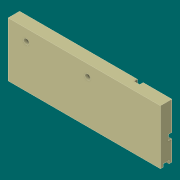
# Autodesk Inventor part: sensorHolder
Saved by Autodesk Inventor 2016 (Build 200138000, 138)
## iProperties
Created: 2015-10-19
Part Number: sensorHolder
Material: ABS Plastic
Document SubType Name: Modeling
Designer: Sawaiz
Density: 1.06 g/cm^3
Appearance: Smooth - Ash
Author: Sawaiz
Autodesk Inventor part; units mm, degrees
ref_plane "YZ Plane" through (0, 0, 0) normal (1, 0, 0) x (0, 1, 0)
ref_plane "XZ Plane" through (0, 0, 0) normal (0, 1, 0) x (-1, 0, 0)
ref_plane "XY Plane" through (0, 0, 0) normal (0, 0, 1) x (1, 0, 0)
sketch "Sketch1" plane through (0, 0, 0) normal (1, 0, 0) x (0, 1, 0)
  line L0 (-57.15, 57.15) -> (57.15, 57.15)
  line L1 (57.15, 57.15) -> (57.15, 0)
  line L2 (57.15, 0) -> (-57.15, 0)
  line L3 (-57.15, 0) -> (-57.15, 57.15)
  line L4 (-57.15, 57.15) -> (57.15, 0) construction
  line L5 (57.15, 57.15) -> (-57.15, 0) construction
  line L6 (-26.9875, 0) -> (26.9875, 0)
  line L7 (26.9875, 0) -> (26.9875, 26.9875)
  line L8 (26.9875, 26.9875) -> (-26.9875, 26.9875)
  line L9 (-26.9875, 26.9875) -> (-26.9875, 0)
  line L10 (-26.9875, 26.9875) -> (-26.9875, 57.15)
  line L11 (26.9875, 26.9875) -> (57.15, 26.9875)
  point P0 (0, 0)
  point P1 (0, 28.575)
  point P2 (0, 0)
  dimension "d5" = 114.3
  dimension "d6" = 57.15
  dimension "d7" = 53.975
  dimension "d8" = 26.9875
  constraints: 24 end point, 4 midpoint, 4 parallel, 3 horizontal, 3 point on line, 2 perpendicular, 1 coincident, 1 vertical
  measures "d5" distance between parallel lines of L3 L1
  measures "d6" distance of L0.end L1.end
  measures "d7" distance of L7.end L8.end
  measures "d8" distance of L6.end L7.end
extrude "Extrusion1" add sketch "Sketch1" along normal blind 6.35 contours L0 L1 L11 L8 L10
sketch "Sketch2" plane through (0, -26.9875, 26.9875) normal (0, 0, -1) x (-1, 0, 0)
  line L0 (0, 0) -> (0, 84.1375) projected
  line L1 (0, 84.1375) -> (-6.35, 84.1375) projected
  line L2 (-6.35, 0) -> (-6.35, 84.1375) projected
  line L3 (0, 0) -> (-6.35, 0) projected
  line L4 (-3.175, 0) -> (-3.175, 84.1375)
  line L5 (-4.7625, 0) -> (-1.5875, 0)
  line L6 (-1.5875, 0) -> (-1.5875, 84.1375)
  line L7 (-1.5875, 84.1375) -> (-4.7625, 84.1375)
  line L8 (-4.7625, 84.1375) -> (-4.7625, 0)
  line L9 (-4.7625, 0) -> (-1.5875, 84.1375) construction
  line L10 (-1.5875, 0) -> (-4.7625, 84.1375) construction
  point P0 (0, 26.9875)
  point P1 (-3.175, 42.0688)
  dimension "d11" = 3.175
  constraints: 14 end point, 5 midpoint, 2 parallel, 1 collinear, 1 horizontal, 1 perpendicular
  measures "d11" distance between parallel lines of L8 L6
extrude "Extrusion2" cut sketch "Sketch2" against normal blind 1.5875 contours L3 L4 L1 L6 | L3 L8 L1 L4
sketch "Sketch3" plane through (6.35, 0, 0) normal (1, 0, 0) x (0, 0, -1)
  line L0 (-26.9875, -26.9875) -> (-26.9875, 57.15) projected
  line L1 (-26.9875, 57.15) -> (-57.15, 57.15) projected
  line L2 (-57.15, 57.15) -> (-57.15, -26.9875) projected
  line L3 (-57.15, -26.9875) -> (-26.9875, -26.9875) projected
  line L4 (-50.8, -16.9333) -> (-50.8, 16.9333)
  point P0 (0, 0)
  dimension "d16" = 40.2167
  dimension "d31" = 33.8667
  dimension "d32" = 6.35
  constraints: 2 end point, 1 vertical
  measures "d16" distance from line of L1 L4.end
  measures "d31" distance of L4.start L4.end
  measures "d32" distance from line of L2 L4.end
hole "Hole1" at (6.35, -16.9333, 50.8) at (6.35, 16.9333, 50.8) direction (-1, 0, 0) diameter 1.778 end through all countersink diameter 3.023 countersink angle 82 clearance for "Flat Head Machine Screw (82)" size "#0" standard "Ansi Unified Screw Threads"
sketch "Sketch4" plane through (0, 0, 0) normal (-1, 0, 0) x (0, 0, 1)
  line L0 (-38.1, -38.1) -> (38.1, -38.1)
  line L1 (38.1, -38.1) -> (38.1, 38.1)
  line L2 (38.1, 38.1) -> (-38.1, 38.1)
  line L3 (-38.1, 38.1) -> (-38.1, -38.1)
  line L4 (-38.1, -38.1) -> (38.1, 38.1) construction
  line L5 (38.1, -38.1) -> (-38.1, 38.1) construction
  line L6 (-41.275, 41.275) -> (41.275, 41.275)
  line L7 (41.275, 41.275) -> (41.275, -41.275)
  line L8 (41.275, -41.275) -> (-41.275, -41.275)
  line L9 (-41.275, -41.275) -> (-41.275, 41.275)
  line L10 (-41.275, 41.275) -> (41.275, -41.275) construction
  line L11 (41.275, 41.275) -> (-41.275, -41.275) construction
  line L12 (26.9875, 57.15) -> (57.15, 57.15) projected
  line L13 (38.1, 38.1) -> (41.275, 38.1)
  line L14 (41.275, 38.1) -> (41.275, 57.15)
  line L15 (41.275, 57.15) -> (38.1, 57.15)
  line L16 (38.1, 57.15) -> (38.1, 38.1)
  line L17 (38.1, 38.1) -> (57.15, 38.1)
  line L18 (57.15, 38.1) -> (57.15, 41.275)
  line L19 (57.15, 41.275) -> (38.1, 41.275)
  line L20 (38.1, 41.275) -> (38.1, 38.1)
  line L21 (57.15, 57.15) -> (57.15, -26.9875) projected
  point P0 (0, 0)
  dimension "d24" = 76.2
  dimension "d25" = 76.2
  dimension "d26" = 3.175
  dimension "d27" = 3.175
  constraints: 40 end point, 8 parallel, 4 horizontal, 4 midpoint, 4 perpendicular, 3 collinear, 1 point on line
  measures "d24" distance of L0.end L1.end
  measures "d25" distance between parallel lines of L3 L1
  measures "d26" distance between parallel lines of L1 L7
  measures "d27" distance between parallel lines of L2 L6
extrude "Extrusion3" cut sketch "Sketch4" against normal blind 1.905 contours L13 L7 L8 L9 L6 L16 | L16 L6 L7 L13 | L7 L19 L18 L17 | L16 L12 L14 L6
equation "\"d5\" = width + 2 * acrylicThickness"
equation "\"d6\" = acrylicThickness + 0.5 * height"
equation "\"d7\" = sensorHolderSensorWidth"
equation "\"d8\" = 0.5 * sensorHolderSesnorHeight"
equation "\"d9\" = acrylicThickness"
equation "\"d11\" = oRingWidth"
equation "\"d12\" = 0.5 * oRingWidth"
equation "\"d16\" = 0.333333 * width + acrylicThickness"
equation "\"d31\" = 0.333333 * width"
equation "\"d32\" = acrylicThickness"
equation "\"d24\" = 0.25 * sensorHolderFlushORingID"
equation "\"d25\" = 0.25 * sensorHolderFlushORingID"
equation "\"d26\" = oRingWidth"
equation "\"d27\" = oRingWidth"
equation "\"acrylicThickness\" = 6.35"
equation "\"height\" = 101.6"
equation "\"width\" = 101.6"
equation "\"depth\" = 101.6"
equation "\"mirrorAngle\" = 5deg"
equation "\"detectorWidth\" = 52"
equation "\"detectorHeight\" = 52"
equation "\"mirrorThickness\" = 3"
equation "\"fresnelThickness\" = 0.1"
equation "\"focalLength\" = 76.2"
equation "\"ior\" = 1.49"
equation "\"centerThickness\" = 1.524"
equation "\"fresnelAngle\" = 90deg"
equation "\"fresnelEffectiveDiameter\" = 76.2"
equation "\"mirrorSuppourtWidth\" = 38.1"
equation "\"backGrooveBit\" = 4.8006"
equation "\"sensorHolderWidth\" = 88.9"
equation "\"sensorHolderHeight\" = 88.9"
equation "\"sensorHolderSesnorHeight\" = 53.975"
equation "\"sensorHolderSensorWidth\" = 53.975"
equation "\"sensorHolderSensorHeight\" = 53.975"
equation "\"sensorHolderORingGroove\" = 3.175"
equation "\"sensorHolderORing\" = 3.175"
equation "\"sensorHolderFlushORing\" = 3.175"
equation "\"sensorHolderFlushORingID\" = 304.8"
equation "\"frontBackORingID\" = 419.1"
equation "\"oRingWidth\" = 3.175"
equation "\"sensorHolderORingID\" = 203.2"
equation "\"topBottomHorizontalMirrorGroove\" = 12.7"
equation "\"backMirrorGroove\" = 6.35"
equation "\"mirrorGroove\" = 19.05"
equation "\"fresnelChamfer\" = 6.35"
equation "\"mirrorGrooveFillet\" = 6.35"
equation "\"mirrorGrooveDrill\" = 6.35"
equation "\"mirrorGrooveMill\" = 3.175"
equation "\"fresnelMirrorChamfer\" = 6.35"
equation "\"detectorOpeningWidth\" = 76.2"
equation "\"detectorOpeningHeight\" = 76.2"
body "Solid1"
